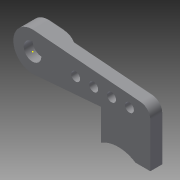
# Autodesk Inventor part: servo_arm_3
Saved by Autodesk Inventor 2015 SP2 (Build 190223200, 223)
## iProperties
Created: 2016-09-12
Part Number: servo_arm_3
Material: Generic
Document SubType Name: Modeling
Designer: jm799
Density: 1 g/cm^3
Appearance: Default
Author: jm799
Autodesk Inventor part; units mm, degrees
ref_plane "YZ Plane" through (0, 0, 0) normal (1, 0, 0) x (0, 1, 0)
ref_plane "XZ Plane" through (0, 0, 0) normal (0, 1, 0) x (-1, 0, 0)
ref_plane "XY Plane" through (0, 0, 0) normal (0, 0, 1) x (1, 0, 0)
sketch "Sketch1" plane through (0, 0, 0) normal (0, 1, 0) x (-1, 0, 0)
  circle A0 centre (0, 0) radius 6.45
  circle A1 centre (0, 0) radius 5.657
  circle A2 centre (0, 0) radius 2.85
  line L0 (0, 0) -> (-36, 0) construction
  circle A3 centre (-36, 0) radius 3.5
  line L1 (0, -6.45) -> (-36, -3.5)
  line L2 (0, 6.45) -> (-36.2847, 3.4884)
  dimension "d0" = 12.9
  dimension "d1" = 11.314
  dimension "d2" = 5.7
  dimension "d3" = 36
  dimension "d4" = 7
  constraints: 6 end point, 4 centre point, 4 coincident, 4 point on circle, 1 horizontal, 1 tangent
  measures "d0" diameter of A0
  measures "d1" diameter of A1
  measures "d2" diameter of A2
  measures "d3" distance of L0.start L0.end
  measures "d4" diameter of A3
extrude "Extrusion1" add sketch "Sketch1" along normal blind 4 contours A0 L1 L2 | A0 L1 A3 L2 | A3 | A1 | A2
sketch "Sketch2" plane through (0, 4, 0) normal (0, 1, 0) x (1, 0, 0)
  circle A0 centre (0, 0) radius 6.45
  line L0 (36, 3.5) -> (0, 6.45) projected
  line L1 (0, -6.45) -> (36.2847, -3.4884) projected
  arc A1 (0, 6.45) -> (0, -6.45) centre (0, 0) ccw
  line L2 (9.9188, -5.6404) -> (9.9188, 5.6372)
  line L3 (9.9188, 5.6372) -> (0, 6.45)
  line L4 (0, -6.45) -> (9.9188, -5.6404)
  dimension "d7" = 12.9
  constraints: 6 end point, 2 centre point, 2 collinear, 2 point on circle, 2 point on line, 1 coincident, 1 vertical
  measures "d7" diameter of A0
extrude "Extrusion2" add sketch "Sketch2" along normal blind 1.5 contours L0 A0 L1 | L0 L2 L1 A0
fillet "Fillet1" radius 10 1 edges at (9.9188, 5.5, 0.0016)
sketch "Sketch3" plane through (0, 5.5, 0) normal (0, 1, 0) x (1, 0, 0)
  circle A0 centre (0, 0) radius 5.657
  dimension "d11" = 11.314
  constraints: 1 centre point, 1 coincident
  measures "d11" diameter of A0
extrude "Extrusion3" cut sketch "Sketch3" against normal blind 1.5
sketch "Sketch4" plane through (0, 4, 0) normal (0, 1, 0) x (1, 0, 0)
  circle A0 centre (0, 0) radius 2.9
  dimension "d14" = 5.8
  constraints: 1 centre point, 1 coincident
  measures "d14" diameter of A0
sketch "Sketch5" plane through (0, 0, 0) normal (0, -1, 0) x (1, 0, 0)
  circle A0 centre (0, 0) radius 2.95
  dimension "d15" = 5.9
  constraints: 1 centre point, 1 coincident
  measures "d15" diameter of A0
extrude "Extrusion4" cut sketch "Sketch5" against normal blind 3
sketch "Sketch6" plane through (0, 4, 0) normal (0, 1, 0) x (1, 0, 0)
  circle A0 centre (0, 0) radius 1.35
  dimension "d18" = 2.7
  constraints: 1 centre point, 1 coincident
  measures "d18" diameter of A0
hole "Hole1" at (0, 4, 0) direction (0, -1, 0) diameter 2.7 end through all
sketch "Sketch7" plane through (0, 0, 0) normal (0, -1, 0) x (1, 0, 0)
  point P0 (0, 0)
sketch "Sketch8" plane through (0, 4, 0) normal (0, 1, 0) x (1, 0, 0)
  line L0 (9.9188, 5.6372) -> (9.9188, -5.6404) construction
  line L1 (9.9188, -0.0016) -> (39.5, -0.0016) construction
  arc A0 (36.2847, -3.4884) -> (36, 3.5) centre (36, 0) ccw construction
  line L2 (32.5, -0.0016) -> (26.5, -0.0016) construction
  circle A1 centre (26.5, -0.0016) radius 1.5 construction
  line L3 (26.5, -0.0016) -> (20.5, -0.0016) construction
  circle A2 centre (20.5, -0.0016) radius 1.5 construction
  circle A3 centre (32.5, -0.0016) radius 1.5 construction
  circle A4 centre (32.5, -0.0016) radius 1.5 construction
  circle A5 centre (32.5, -0.0016) radius 1.5
  circle A6 centre (26.5, -0.0016) radius 1.5
  circle A7 centre (20.5, -0.0016) radius 1.5
  point P0 (0, 0)
  dimension "d27" = 6
  dimension "d28" = 3
  dimension "d29" = 6
  dimension "d30" = 3
  dimension "d31" = 3
  dimension "d32" = 3
  dimension "d33" = 3
  dimension "d34" = 3
  constraints: 7 centre point, 7 coincident, 6 end point, 3 point on line, 1 midpoint, 1 perpendicular, 1 point on circle
  measures "d27" distance of L2.start L2.end
  measures "d28" diameter of A1
  measures "d29" distance of L3.start L3.end
  measures "d30" diameter of A2
  measures "d31" diameter of A4
  measures "d32" diameter of A5
  measures "d33" diameter of A6
  measures "d34" diameter of A7
hole "Hole2" at (20.5, 4, 0.0016) at (26.5, 4, 0.0016) at (32.5, 4, 0.0016) direction (0, -1, 0) diameter 3 end through all
sketch "Sketch9" plane through (0, 4, 0) normal (0, 1, 0) x (1, 0, 0)
  arc A0 (36.2847, -3.4884) -> (36, 3.5) centre (36, 0) ccw projected
  line L0 (39.5, 0) -> (39.5, 15)
  line L1 (39.5, 15) -> (22.9619, 15)
  line L2 (22.9619, 15) -> (22.9619, 4.5684)
  line L3 (36, 3.5) -> (0, 6.45) projected
  point P0 (0, 0)
  dimension "d46" = 15
  constraints: 6 end point, 2 perpendicular, 1 point on circle, 1 point on line, 1 tangent, 1 vertical
  measures "d46" distance of L0.start L0.end
extrude "Extrusion5" add sketch "Sketch9" against normal blind 4
sketch "Sketch10" plane through (0, 4, 0) normal (0, 1, 0) x (1, 0, 0)
  line L0 (39.5, 15) -> (22.9619, 15)
  line L1 (22.9619, 15) -> (39.5, 15) projected
  line L2 (22.9619, 15) -> (39.5, 15) projected
  arc A0 (23.6935, 15) -> (35.6591, 15) centre (29.6763, 28.5077) ccw
  point P0 (0, 0)
  constraints: 2 end point, 2 point on circle, 2 point on line, 1 centre point, 1 collinear
extrude "Extrusion6" [suppressed]
sketch "Sketch11" plane through (0, 4, 0) normal (0, 1, 0) x (1, 0, 0)
  circle A0 centre (20.5, -0.0016) radius 1.5 construction
  line L0 (19, -0.0016) -> (16, -0.0016) construction
  circle A1 centre (14.4602, -0.0016) radius 1.5 construction
  circle A2 centre (14.4602, -0.0016) radius 1.5
  point P0 (0, 0)
  dimension "d47" = 3
  dimension "d48" = 3
  constraints: 2 centre point, 2 end point, 1 coincident, 1 concentric, 1 horizontal, 1 horizontal alignment, 1 other
  measures "d47" distance of L0.start L0.end
  measures "d48" diameter of A1
hole "Hole3" at (14.4602, 4, 0.0016) direction (0, -1, 0) diameter 3 end through all
sketch "Sketch12" plane through (0, 4, 0) normal (0, 1, 0) x (1, 0, 0)
  line L0 (39.5, 15) -> (22.9619, 15)
  line L1 (22.9619, 15) -> (39.5, 15) projected
  arc A0 (22.9619, 15) -> (34.5413, 15) centre (28.7516, 24.0306) ccw
  point P0 (0, 0)
  constraints: 2 end point, 2 point on circle, 1 centre point, 1 horizontal, 1 point on line
extrude "Extrusion7" cut sketch "Sketch12" against normal blind 4
body "Solid1"
